lead_screw_for_3d_v7 (Autodesk Fusion 360 design; units mm, degrees)
Autodesk Fusion 360 part; units mm, degrees
note: some values were not read from the file. Set by a fixed rule: which sketch regions a step uses.
sketch "Sketch1" plane through (0, 0, 0) normal (0, 1, 0) x (1, 0, 0)
  line L0 (0, 0) -> (115, 0)
  line L1 (115, -36) -> (0, -36)
  circle A0 centre (5.75, -26) radius 2.15
  circle A1 centre (5.75, -5) radius 2.15
  circle A2 centre (33.75, -5) radius 2.15
  circle A3 centre (33.75, -26) radius 2.15
  circle A4 centre (81.25, -5) radius 2.15
  circle A5 centre (81.25, -26) radius 2.15
  circle A6 centre (109.25, -5.0525) radius 2.15
  circle A7 centre (109.25, -26.0525) radius 2.15
  line L2 (73.45, -36) -> (73.45, 0) construction
  line L3 (41.55, -36) -> (41.55, 0) construction
  line L4 (5.75, -26) -> (39, -26) construction
  line L5 (0, 0) -> (-2.05, 0)
  line L6 (-2.05, 0) -> (-2.05, -36)
  line L7 (-2.05, -36) -> (0, -36)
  line L8 (115, 0) -> (117.05, 0)
  line L9 (117.05, 0) -> (117.05, -36)
  line L10 (117.05, -36) -> (115, -36)
  dimension "d1" = 115
  dimension "d2" = 36
  dimension "d3" = 4.3
  dimension "d4" = 4.3
  dimension "d7" = 21
  dimension "d8" = 5
  dimension "d13" = 4.3
  dimension "d14" = 4.3
  dimension "d15" = 21
  dimension "d16" = 4.3
  dimension "d17" = 4.3
  dimension "d18" = 21
  dimension "d19" = 4.3
  dimension "d20" = 4.3
  dimension "d21" = 21
  dimension "d40" = 28
  dimension "d41" = 28
  dimension "d44" = 28
  dimension "d45" = 28
  dimension "d46" = 5
  dimension "d47" = 7.8
  dimension "d48" = 7.8
  dimension "d50" = 7.8
  dimension "d51" = 7.8
  constraint horizontal L0
  constraint horizontal L1
  constraint coincident L0.start L5.start
  constraint coincident L1 L2.start
  constraint perpendicular L1 L2
  constraint coincident L1 L3.start
  constraint coincident L0 L3.end
  constraint perpendicular L0 L3
  constraint coincident A0.centre L4.start
  constraint parallel L1 L4
  constraint coincident A3.centre L4
  constraint perpendicular L1 L6
  constraint perpendicular L1 L9
  measures "d1" distance of L0.start L0.end
  measures "d2" distance of L0.start L1.end
  measures "d3" diameter of A0
  measures "d4" diameter of A1
  measures "d7" distance of A0.centre A1.centre
  measures "d8" distance of L0 A1.centre
  measures "d13" diameter of A3
  measures "d14" diameter of A2
  measures "d15" distance of A2.centre A3.centre
  measures "d16" diameter of A5
  measures "d17" diameter of A4
  measures "d18" distance of A4.centre A5.centre
  measures "d19" diameter of A7
  measures "d20" diameter of A6
  measures "d21" distance of A7.centre A6.centre
  measures "d40" distance of A0.centre A3.centre
  measures "d41" horizontal distance of A1.centre A2.centre
  measures "d44" distance of A5.centre A7.centre
  measures "d45" horizontal distance of A4.centre A6.centre
  measures "d46" distance of L0 A4.centre
  measures "d47" distance of A2.centre L3
  measures "d48" distance of A4.centre L2
  measures "d50" distance of A1.centre L6
  measures "d51" distance of A6.centre L9
extrude "Extrude1" add sketch "Sketch1" along normal blind 8
sketch "Sketch2" plane through (0, 0, 36) normal (0, 0, 1) x (1, 0, 0)
  line L0 (-2.05, 0) -> (117.05, 0)
  line L1 (117.05, 8) -> (-2.05, 8)
  line L2 (45, 8) -> (70, 8)
  line L3 (70, 8) -> (70, -8)
  line L4 (70, -8) -> (45, -8)
  line L5 (45, -8) -> (45, 8)
  line L6 (45, 8) -> (70, -8) construction
  line L7 (70, 8) -> (45, -8) construction
  circle A0 centre (57.5, -27.1) radius 11
  circle A1 centre (57.5, -27.1) radius 5.4
  circle A2 centre (57.5, -27.1) radius 8
  line L8 (65.5, -27.1) -> (49.5, -27.1) construction
  line L9 (57.5005, -35.1) -> (57.5005, -19.1) construction
  circle A3 centre (65.5, -27.1) radius 2.05
  circle A4 centre (57.5005, -35.1) radius 2.05
  circle A5 centre (49.5, -27.1) radius 2.05
  circle A6 centre (57.5005, -19.1) radius 2.05
  line L10 (70, -8) -> (45, -8)
  line L11 (45, -8) -> (45, -41)
  line L12 (45, -41) -> (70, -41)
  line L13 (70, -41) -> (70, -8)
  line L14 (115, 0) -> (0, 0)
  line L15 (117.05, 0) -> (117.05, 8)
  line L16 (-2.05, 8) -> (-2.05, 0)
  point P0 (57.5, 0)
  dimension "d26" = 25
  dimension "d27" = 16
  dimension "d28" = 22
  dimension "d29" = 10.8
  dimension "d30" = 16
  dimension "d31" = 4.1
  dimension "d32" = 4.1
  dimension "d33" = 4.1
  dimension "d34" = 4.1
  dimension "d35" = 33
  dimension "d39" = 27.1
  constraint horizontal L2
  constraint perpendicular L2 L3
  constraint parallel L2 L4
  constraint parallel L3 L5
  constraint coincident L6 P0
  constraint coincident L7 P0
  constraint midpoint L0 P0
  constraint concentric A0 A1
  constraint concentric A1 A2
  constraint coincident A2 L8.start
  constraint coincident A2 L8.end
  constraint horizontal L8
  constraint coincident A2 L9.start
  constraint coincident A2 L9.end
  constraint perpendicular L8 L9
  constraint vertical P0 A0.centre
  constraint coincident L8.start A3.centre
  constraint coincident L9.start A4.centre
  constraint coincident L8.end A5.centre
  constraint coincident L9.end A6.centre
  constraint horizontal L10
  constraint vertical L11
  constraint horizontal L12
  constraint vertical L13
  measures "d26" distance of L3.end L4.end
  measures "d27" distance of L2.end L3.end
  measures "d28" diameter of A0
  measures "d29" diameter of A1
  measures "d30" diameter of A2
  measures "d31" diameter of A3
  measures "d32" diameter of A4
  measures "d33" diameter of A5
  measures "d34" diameter of A6
  measures "d35" distance of L3.end L12.end
  measures "d39" distance of A0.centre L14
extrude "Extrude2" add sketch "Sketch2" against normal blind 12 from surface at -14 contours L0 L3 L4 L5 L10 L14 | L4 L10 L11 L12 L13 | A0 | A2 A3 A4 A5 A6
chamfer "Chamfer2" distance 5 angle 45 2 edges at (57.5, 0, 22) (57.5, 0, 10)
extrude "Extrude3" cut sketch "Sketch2" against normal blind 16 contours A0 | A2 A3 A4 A5 A6
extrude "Extrude4" cut sketch "Sketch2" along normal blind 2 from surface at -27 contours A0 | A2 A3 A4 A5 A6
extrude "Extrude5" add 1 faces at (64.771, 8, 18.689) along direction (0, 1, 0) blind 4
sketch "Sketch3" plane through (0, 12, 0) normal (0, 1, 0) x (-1, 0, 0)
  circle A0 centre (-109.25, 5.0525) radius 2.15
  circle A1 centre (-33.75, 26) radius 2.15
  circle A2 centre (-81.25, 26) radius 2.15
  circle A3 centre (-5.75, 5) radius 2.15
  circle A4 centre (-109.25, 26.0525) radius 2.15
  circle A5 centre (-5.75, 26) radius 2.15
  circle A6 centre (-81.25, 5) radius 2.15
  circle A7 centre (-33.75, 5) radius 2.15
  line L0 (-117.05, 0) -> (2.05, 0)
  line L1 (2.05, 0) -> (2.05, 36)
  line L2 (2.05, 36) -> (-117.05, 36)
  line L3 (-117.05, 36) -> (-117.05, 0)
  circle A8 centre (-81.25, 5) radius 4.75
  circle A9 centre (-81.25, 26) radius 4.75
  circle A10 centre (-109.25, 26.0525) radius 4.75
  circle A11 centre (-109.25, 5.0525) radius 4.75
  circle A12 centre (-33.75, 26) radius 4.75
  circle A13 centre (-5.75, 26) radius 4.75
  circle A14 centre (-33.75, 5) radius 4.75
  circle A15 centre (-5.75, 5) radius 4.75
  dimension "d60" = 9.5
  dimension "d61" = 9.5
  dimension "d62" = 9.5
  dimension "d63" = 9.5
  dimension "d64" = 9.5
  dimension "d65" = 9.5
  dimension "d66" = 9.5
  dimension "d67" = 9.5
  constraint concentric A6 A8
  constraint concentric A2 A9
  constraint concentric A4 A10
  constraint concentric A0 A11
  constraint concentric A1 A12
  constraint concentric A5 A13
  constraint concentric A7 A14
  constraint concentric A3 A15
  measures "d60" diameter of A8
  measures "d61" diameter of A9
  measures "d62" diameter of A10
  measures "d63" diameter of A11
  measures "d64" diameter of A12
  measures "d65" diameter of A13
  measures "d66" diameter of A14
  measures "d67" diameter of A15
extrude "Extrude6" add sketch "Sketch3" along normal blind 50 contours L0 L1 L2 L3
extrude "Extrude7" add 1 faces at (37.65, 41.3333, 0) along direction (0, 0, -1) blind 5
chamfer "Chamfer3" distance 5 angle 45 2 edges at (45, 0, 16) (70, 0, 16)
sketch "Sketch4" plane through (0, 0, -5) normal (0, 0, -1) x (-1, 0, 0)
  line L0 (-117.05, 0) -> (2.05, 0)
  line L1 (2.05, 0) -> (2.05, 62)
  line L2 (2.05, 62) -> (-117.05, 62)
  line L3 (-117.05, 62) -> (-117.05, 0)
  line L4 (-77.5, 32) -> (-37.5, 32)
  line L5 (-37.5, 32) -> (-37.5, 28)
  line L6 (-37.5, 28) -> (-77.5, 28)
  line L7 (-77.5, 28) -> (-77.5, 32)
  line L8 (-57.5, 62) -> (-57.5, 32) construction
  line L9 (-57.5, 28) -> (-57.5, 0) construction
  dimension "d73" = 40
  dimension "d74" = 4
  dimension "d75" = 30
  dimension "d78" = 20
  constraint midpoint L2 L8.start
  constraint midpoint L0 L9.end
  constraint horizontal L4
  constraint perpendicular L4 L5
  constraint parallel L4 L6
  constraint parallel L5 L7
  constraint coincident L4 L8.end
  constraint coincident L6 L9.start
  constraint collinear L8 L9
  measures "d73" distance of L5.end L6.end
  measures "d74" distance of L4.end L5.end
  measures "d75" distance of L2 L4
  measures "d78" distance of L5.end L9.start
extrude "Extrude8" cut sketch "Sketch4" against normal blind 50 contours L4 L5 L6 L7
